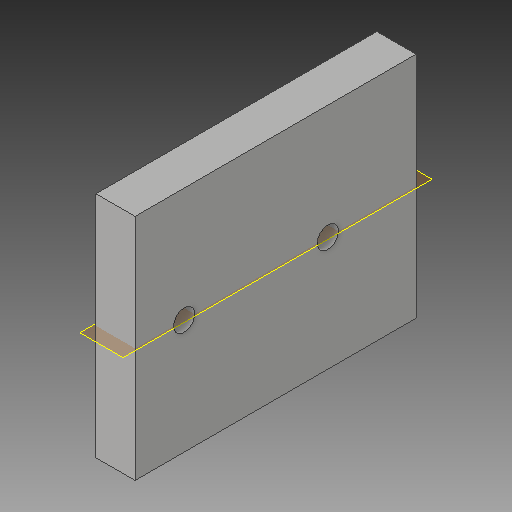
# Autodesk Inventor part: MotorHolderLongAxisBottom
Saved by Autodesk Inventor 2018 (Build 220112000, 112)
## iProperties
Created: 2017-10-24
Part Number: MotorHolderLongAxisBottom
Material: Generic
Document SubType Name: Modeling
Designer: m228540
Density: 1 g/cm^3
Appearance: Default
Mass: 70.5954 g
Surface Area: 167.068 cm^2
Volume: 70.5954 cm^3
Author: m228540
Autodesk Inventor part; units mm, degrees
ref_plane "YZ Plane" through (0, 0, 0) normal (1, 0, 0) x (0, 1, 0)
ref_plane "XZ Plane" through (0, 0, 0) normal (0, 1, 0) x (-1, 0, 0)
ref_plane "XY Plane" through (0, 0, 0) normal (0, 0, 1) x (1, 0, 0)
sketch "Sketch1" plane through (0, 0, 0) normal (1, 0, 0) x (0, 1, 0)
  line L0 (-35, 43) -> (35, 43)
  line L1 (35, 43) -> (35, -43)
  line L2 (35, -43) -> (-35, -43)
  line L3 (-35, -43) -> (-35, 43)
  line L4 (-35, 43) -> (35, -43) construction
  line L5 (35, 43) -> (-35, -43) construction
  point P0 (0, 0)
  dimension "d0" = 86
  dimension "d1" = 70
  constraints: 12 end point, 2 midpoint, 2 parallel, 1 horizontal, 1 perpendicular
  measures "d0" distance of L0.end L1.end
  measures "d1" distance of L0.start L0.end
extrude "Extrusion1" add sketch "Sketch1" along normal blind 12
ref_plane "Work Plane1" through (0, 0, 43) normal (0, 1, 0) x (1, 0, 0)
sketch "Sketch2" plane through (0, -35, -43) normal (0, 0, -1) x (-1, 0, 0)
  circle A0 centre (-6, 60) radius 3
  circle A1 centre (-6, 35) radius 3 construction
  circle A2 centre (-6, 10) radius 3
  line L0 (0, 70) -> (-12, 70) projected
  line L1 (-6, 70) -> (-6, 0) construction
  line L2 (0, 0) -> (-12, 0) projected
  point P0 (0, 35)
  dimension "d4" = 6
  dimension "d5" = 25
  dimension "d6" = 25
  constraints: 4 midpoint, 3 centre point, 2 end point, 2 equal radius, 2 point on line
  measures "d4" diameter of A1
  measures "d5" distance of A0.centre A1.centre
  measures "d6" distance of A2.centre A1.centre
extrude "Extrusion2" cut sketch "Sketch2" against normal blind 15
sketch "Sketch3" plane through (12, 0, 0) normal (1, 0, 0) x (0, 0, -1)
  circle A0 centre (-46.1752, 0) radius 3 projected
  circle A1 centre (-111.1482, 0) radius 3 projected
  circle A2 centre (-90.1752, 0) radius 3 projected
  point P0 (0, 0)
extrude "Extrusion3" cut sketch "Sketch3" against normal through all
sketch "Sketch4" plane through (0, 0, 0) normal (-1, 0, 0) x (0, 0, 1)
  circle A0 centre (28, 0) radius 3 construction
  circle A1 centre (-16, 0) radius 3 construction
  circle A2 centre (28, 0) radius 3.25
  circle A3 centre (-16, 0) radius 3.25
  point P0 (0, 0)
  dimension "d13" = 0.25
  dimension "d14" = 0.25
  constraints: 2 centre point
  measures "d13" radial gap between concentric circles of A0 A2
  measures "d14" radial gap between concentric circles of A1 A3
extrude "Extrusion4" cut sketch "Sketch4" against normal through all
thread "Thread1" size "M6x1" class "6H" standard "ANSI Metric M Profile" full length
thread "Thread2" size "M6x1" class "6H" standard "ANSI Metric M Profile" full length
body "Solid1"
